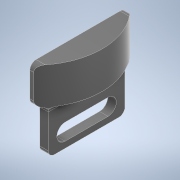
# Autodesk Inventor part: yystop
Saved by Autodesk Inventor 2022 (Build 260153000, 153)
## iProperties
Created: 2022-07-18
Part Number: yystop
Material: Genérico
Document SubType Name: Modeling
Designer: JK
Density: 1 g/cm^3
Appearance: Suave - Negro
Author: JK
Autodesk Inventor part; units mm, degrees
ref_plane "YZ Plane" through (0, 0, 0) normal (1, 0, 0) x (0, 1, 0)
ref_plane "XZ Plane" through (0, 0, 0) normal (0, 1, 0) x (-1, 0, 0)
ref_plane "XY Plane" through (0, 0, 0) normal (0, 0, 1) x (1, 0, 0)
sketch "Boceto1" plane through (0, 0, 0) normal (0, 1, 0) x (-1, 0, 0)
  line L0 (-14.8958, 23.7803) -> (7.8042, 23.7803)
  line L1 (7.8042, 23.7803) -> (7.8042, -7.6197)
  line L2 (7.8042, -7.6197) -> (-14.8958, -7.6197)
  line L3 (-14.8958, -7.6197) -> (-14.8958, 23.7803)
  line L4 (-14.8958, 23.7803) -> (7.8042, -7.6197) construction
  line L5 (7.8042, 23.7803) -> (-14.8958, -7.6197) construction
  arc A0 (-14.8958, 23.7803) -> (-14.8958, -7.6197) centre (0.5156, 8.0803) ccw
  line L6 (7.8042, 17.8112) -> (7.8042, 23.7803)
  line L7 (-13.6958, 20.5803) -> (6.6042, 20.5803)
  line L8 (6.6042, 20.5803) -> (6.6042, -4.4197)
  line L9 (6.6042, -4.4197) -> (-13.6958, -4.4197)
  line L10 (-13.6958, -4.4197) -> (-13.6958, 20.5803)
  line L11 (-13.6958, 20.5803) -> (6.6042, -4.4197) construction
  line L12 (6.6042, 20.5803) -> (-13.6958, -4.4197) construction
  line L13 (7.8042, 23.7803) -> (11.6042, 23.7803)
  line L14 (11.6042, 23.7803) -> (11.6042, -7.6197)
  line L15 (11.6042, -7.6197) -> (7.8042, -7.6197)
  line L16 (7.8042, -7.6197) -> (7.8042, 23.7803)
  line L17 (7.8042, 23.7803) -> (6.6042, 23.7803)
  line L18 (6.6042, 23.7803) -> (6.6042, -7.6197)
  line L19 (6.6042, -7.6197) -> (7.8042, -7.6197)
  line L20 (7.8042, -7.6197) -> (7.8042, 23.7803)
  line L21 (11.6042, -7.6197) -> (6.6042, -7.6197)
  line L22 (6.6042, -7.6197) -> (6.6042, -4.4197)
  line L23 (6.6042, -4.4197) -> (11.6042, -4.4197)
  line L24 (11.6042, -4.4197) -> (11.6042, -7.6197)
  line L25 (11.6042, 23.7803) -> (6.6042, 23.7803)
  line L26 (6.6042, 23.7803) -> (6.6042, 20.5803)
  line L27 (6.6042, 20.5803) -> (11.6042, 20.5803)
  line L28 (11.6042, 20.5803) -> (11.6042, 23.7803)
  line L29 (-14.8958, 23.7803) -> (-13.6958, 23.7803)
  line L30 (-13.6958, 23.7803) -> (-13.6958, -7.6197)
  line L31 (-13.6958, -7.6197) -> (-14.8958, -7.6197)
  line L32 (-14.8958, -7.6197) -> (-14.8958, 23.7803)
  point P0 (-3.5458, 8.0803)
  point P1 (6.6042, -4.4197)
  point P2 (6.6042, 20.5803)
  point P3 (6.6042, 23.7803)
  point P4 (6.6042, 20.5803)
  point P5 (11.6042, -4.4197)
  point P6 (6.6042, -4.4197)
  dimension "d4" = 25
  dimension "d5" = 3.2
  dimension "d6" = 1.2
  dimension "d7" = 20.3
  dimension "d14" = 5
  dimension "d34" = 22
  constraints: 66 end point, 14 parallel, 7 horizontal, 7 perpendicular, 4 midpoint, 4 point on line, 2 point on circle, 1 centre point
  measures "d4" distance of L7.end L8.end
  measures "d5" distance between parallel lines of L7 L0
  measures "d6" distance between parallel lines of L10 L3
  measures "d7" distance of L7.start L7.end
  measures "d14" distance between parallel lines of L14 L18
  measures "d34" radius of A0
extrude "Extrusión1" add sketch "Boceto1" along normal blind 12 contours L0 L30 L10 L2 L3 | L3 A0
sketch "Boceto3" plane through (0, 0, 0) normal (0, -1, 0) x (1, 0, 0)
  line L0 (10.8958, -4.4197) -> (16.4958, -4.4197)
  line L1 (16.4958, -4.4197) -> (16.4958, 20.5803)
  line L2 (16.4958, 20.5803) -> (10.8958, 20.5803)
  line L3 (10.8958, 20.5803) -> (10.8958, -4.4197)
  line L4 (13.6958, -7.6197) -> (13.6958, 23.7803) projected
  line L5 (10.8958, -4.4197) -> (16.4958, 20.5803) construction
  line L6 (16.4958, -4.4197) -> (10.8958, 20.5803) construction
  point P0 (0, 0)
  point P1 (13.6958, 8.0803)
  point P2 (13.6958, 20.5803)
  point P3 (13.6958, -4.4197)
  dimension "d18" = 25
  dimension "d19" = 2.8
  constraints: 12 end point, 3 midpoint, 2 parallel, 1 horizontal, 1 perpendicular
  measures "d18" distance of L2.end L0.start
  measures "d19" distance between parallel lines of L4 L1
extrude "Extrusión3" add sketch "Boceto3" along normal blind 15 contours L4 L2 L1 L0
fillet "Empalme2" radius 2 9 edges at (15.0958, 0, 20.5803) (15.0958, -15, 20.5803) (15.0958, -15, -4.4197) (15.0958, 0, -4.4197) (14.2958, 0, -7.6197) (14.2958, 12, -7.6197) (14.2958, 0, 23.7803) (14.2958, 12, 23.7803) (16.4958, 0, 8.0803)
sketch "Boceto4" plane through (16.4958, -13, -4.4197) normal (1, 0, 0) x (0, 0, -1)
  circle A0 centre (-19.5, 2.7) radius 2.7
  circle A1 centre (-5.5, 2.7) radius 2.7
  line L0 (-19.5, 5.4) -> (-5.5, 5.4)
  line L1 (-5.5, 5.4) -> (-5.5, 0)
  line L2 (-5.5, 0) -> (-19.5, 0)
  line L3 (-19.5, 0) -> (-19.5, 5.4)
  line L4 (-25, 11) -> (-25, 0) projected
  line L5 (0, 11) -> (0, 0) projected
  line L6 (-2, -2) -> (-23, -2) projected
  point P0 (-4.4197, 13)
  point P1 (-5.5, 0)
  point P2 (-5.5, 5.4)
  point P3 (-19.5, 5.4)
  dimension "d23" = 5.4
  dimension "d24" = 5.5
  dimension "d25" = 5.5
  dimension "d26" = 2
  constraints: 8 end point, 4 tangent, 2 centre point, 2 midpoint, 2 parallel, 1 horizontal, 1 perpendicular
  measures "d23" diameter of A0
  measures "d24" distance from line of L4 A0.centre
  measures "d25" distance from line of L5 A1.centre
  measures "d26" distance between parallel lines of L2 L6
extrude "Extrusión4" cut sketch "Boceto4" against normal through all
sketch "Boceto5" plane through (16.4958, -13, -4.4197) normal (1, 0, 0) x (0, 0, -1)
  arc A0 (-5.5, 0) -> (-5.5, 5.4) centre (-5.5, 2.7) ccw projected
  line L0 (-5.5, 0) -> (-19.5, 0) projected
  arc A1 (-19.5, 5.4) -> (-19.5, 0) centre (-19.5, 2.7) ccw projected
  line L1 (-19.5, 5.4) -> (-5.5, 5.4) projected
  arc A2 (-2, -2) -> (0, 0) centre (-2, 0) ccw projected
  line L2 (0, 11) -> (0, 0) projected
  line L3 (-25, 11) -> (0, 11) projected
  line L4 (-25, 11) -> (-25, 0) projected
  arc A3 (-25, 0) -> (-23, -2) centre (-23, 0) ccw projected
  line L5 (-2, -2) -> (-23, -2) projected
  arc A4 (-5.5, -2) -> (-5.5, 7.4) centre (-5.5, 2.7) ccw
  line L6 (-5.5, -2) -> (-19.5, -2)
  arc A5 (-19.5, 7.4) -> (-19.5, -2) centre (-19.5, 2.7) ccw
  line L7 (-19.5, 7.4) -> (-5.5, 7.4)
  point P0 (-4.4197, 13)
  point P1 (-21.3974, 7)
  point P2 (-19.5, -2)
  point P3 (-5.5, -2)
  point P4 (-3.6026, 7)
  dimension "d29" = 2
  constraints: 4 end point, 4 point on circle, 2 centre point, 3 other
  measures "d29" distance between parallel lines of L1 L7
sketch "Boceto2" plane through (-6.6042, 0, 23.7803) normal (0, 0, 1) x (1, 0, 0)
  circle A0 centre (2.3, 6) radius 2.7
  line L0 (-5, 0) -> (21.5, 0) projected
  circle A1 centre (10.3, 6) radius 2.7
  line L1 (2.3, 3.3) -> (10.3, 3.3)
  line L2 (10.3, 3.3) -> (10.3, 8.7)
  line L3 (10.3, 8.7) -> (2.3, 8.7)
  line L4 (2.3, 8.7) -> (2.3, 3.3)
  point P0 (6.6042, 0)
  point P1 (20.3, 0)
  dimension "d10" = 5.4
  dimension "d11" = 6
  dimension "d12" = 10
  dimension "d13" = 8
  constraints: 8 end point, 2 horizontal, 2 parallel, 2 tangent, 1 centre point, 1 perpendicular, 1 vertical alignment, 3 other
  measures "d11" distance from line of L0 point (2.3, 6)
  measures "d12" horizontal distance of point (20.3, 0) A1.centre
  measures "d13" distance of L1.start L1.end
